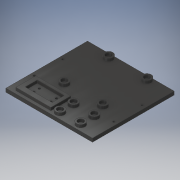
# Autodesk Inventor part: circuirt_board
Saved by Autodesk Inventor 2019 (Build 230136000, 136)
## iProperties
Created: 2018-11-27
Part Number: circuirt_board
Material: Generic
Document SubType Name: Modeling
Designer: xwermter
Density: 1 g/cm^3
Appearance: Default
Author: xwermter
Autodesk Inventor part; units mm, degrees
ref_plane "YZ Plane" through (0, 0, 0) normal (1, 0, 0) x (0, 1, 0)
ref_plane "XZ Plane" through (0, 0, 0) normal (0, 1, 0) x (-1, 0, 0)
ref_plane "XY Plane" through (0, 0, 0) normal (0, 0, 1) x (1, 0, 0)
sketch "Sketch1" plane through (0, 0, 0) normal (0, 1, 0) x (-1, 0, 0)
  line L0 (60.75, -57.25) -> (-60.75, -57.25)
  line L1 (-60.75, -57.25) -> (-60.75, 57.25)
  line L2 (-60.75, 57.25) -> (60.75, 57.25)
  line L3 (60.75, 57.25) -> (60.75, -57.25)
  line L4 (0, -80.15) -> (0, 80.15) projected
  line L5 (-85.05, 0) -> (85.05, 0) projected
  dimension "d0" = 121.5
  dimension "d1" = 114.5
  constraints: 8 end point, 2 parallel, 1 horizontal, 1 perpendicular, 2 other
  measures "d0" distance of L1.end L2.end
  measures "d1" distance of L0.end L1.end
extrude "Extrusion1" add sketch "Sketch1" along normal blind 5
sketch "Sketch3" plane through (0, 5, 0) normal (0, 1, 0) x (1, 0, 0)
  circle A0 centre (-36.75, -34.25) radius 1.5
  line L0 (-60.75, 57.25) -> (-60.75, -57.25) projected
  circle A1 centre (-12.75, -34.25) radius 1.5
  circle A2 centre (-36.75, -42.25) radius 1.5
  circle A3 centre (-12.75, -42.25) radius 1.5
  line L1 (-60.75, -57.25) -> (60.75, -57.25) projected
  circle A4 centre (-55.75, -22.25) radius 1.5
  circle A5 centre (-55.75, 17.75) radius 1.5
  circle A6 centre (-25.25, 51.25) radius 1.5
  circle A7 centre (28.75, 51.25) radius 1.5
  circle A8 centre (55.75, 17.75) radius 1.5
  circle A9 centre (55.75, -22.25) radius 1.5
  line L2 (60.75, 57.25) -> (-60.75, 57.25) projected
  line L3 (60.75, -57.25) -> (60.75, 57.25) projected
  circle A10 centre (-25.25, -10.75) radius 1.5
  circle A11 centre (28.75, -10.75) radius 1.5
  circle A12 centre (6.75, -29.75) radius 1.5
  circle A13 centre (6.75, -48.75) radius 1.5
  circle A14 centre (35.75, -48.75) radius 1.5
  circle A15 centre (35.75, -29.75) radius 1.5
  point P0 (0, 0)
  dimension "d11" = 3
  dimension "d12" = 24
  dimension "d13" = 3
  dimension "d14" = 3
  dimension "d15" = 3
  dimension "d16" = 24
  dimension "d17" = 24
  dimension "d20" = 23
  dimension "d21" = 23
  dimension "d22" = 8
  dimension "d23" = 8
  dimension "d24" = 15
  dimension "d25" = 3
  dimension "d26" = 3
  dimension "d27" = 5
  dimension "d28" = 5
  dimension "d29" = 35
  dimension "d30" = 40
  dimension "d31" = 3
  dimension "d32" = 3
  dimension "d33" = 3
  dimension "d34" = 3
  dimension "d35" = 6
  dimension "d36" = 6
  dimension "d37" = 5
  dimension "d38" = 5
  dimension "d39" = 35
  dimension "d40" = 40
  dimension "d41" = 32
  dimension "d42" = 54
  dimension "d43" = 3
  dimension "d44" = 3
  dimension "d45" = 62
  dimension "d46" = 62
  dimension "d47" = 54
  dimension "d48" = 32
  dimension "d49" = 3
  dimension "d50" = 3
  dimension "d51" = 3
  dimension "d52" = 3
  dimension "d53" = 8.5
  dimension "d54" = 8.5
  dimension "d55" = 25
  dimension "d56" = 29
  dimension "d57" = 19
  dimension "d58" = 19
  dimension "d59" = 25
  dimension "d60" = 29
  constraints: 16 centre point
  measures "d11" diameter of A0
  measures "d12" distance from line of L0 A0.centre
  measures "d13" diameter of A1
  measures "d14" diameter of A2
  measures "d15" diameter of A3
  measures "d16" distance of A1.centre A0.centre
  measures "d17" distance of A3.centre A2.centre
  measures "d20" distance from line of L1 A0.centre
  measures "d21" distance from line of L1 A1.centre
  measures "d22" distance of A0.centre A2.centre
  measures "d23" distance of A1.centre A3.centre
  measures "d24" distance from line of L1 A2.centre
  measures "d25" diameter of A4
  measures "d26" diameter of A5
  measures "d27" distance from line of L0 A5.centre
  measures "d28" distance from line of L0 A4.centre
  measures "d29" distance from line of L1 A4.centre
  measures "d30" distance of A4.centre A5.centre
  measures "d31" diameter of A6
  measures "d32" diameter of A7
  measures "d33" diameter of A8
  measures "d34" diameter of A9
  measures "d35" distance from line of L2 A6.centre
  measures "d36" distance from line of L2 A7.centre
  measures "d37" distance from line of L3 A8.centre
  measures "d38" distance from line of L3 A9.centre
  measures "d39" distance from line of L1 A9.centre
  measures "d40" distance of A8.centre A9.centre
  measures "d41" distance from line of L3 A7.centre
  measures "d42" distance of A6.centre A7.centre
  measures "d43" diameter of A10
  measures "d44" diameter of A11
  measures "d45" distance of A6.centre A10.centre
  measures "d46" distance of A11.centre A7.centre
  measures "d47" distance of A11.centre A10.centre
  measures "d48" distance from line of L3 A11.centre
  measures "d49" diameter of A12
  measures "d50" diameter of A13
  measures "d51" diameter of A14
  measures "d52" diameter of A15
  measures "d53" distance from line of L1 A13.centre
  measures "d54" distance from line of L1 A14.centre
  measures "d55" distance from line of L3 A14.centre
  measures "d56" distance of A13.centre A14.centre
  measures "d57" distance of A13.centre A12.centre
  measures "d58" distance of A14.centre A15.centre
  measures "d59" distance from line of L3 A15.centre
  measures "d60" distance of A15.centre A12.centre
extrude "Extrusion2" cut sketch "Sketch3" against normal through all contours A0 | A1 | A2 | A3 | A4 | A5 | A6 | A7 | A8 | A9 | A10 | A11 | A12 | A13 | A14 | A15
sketch "Sketch4" plane through (0, 5, 0) normal (0, 1, 0) x (1, 0, 0)
  line L0 (-44.75, -29.25) -> (-6.75, -29.25)
  line L1 (-6.75, -29.25) -> (-6.75, -46.25)
  line L2 (-6.75, -46.25) -> (-44.75, -46.25)
  line L3 (-44.75, -46.25) -> (-44.75, -29.25)
  line L4 (-50.75, -25.25) -> (-1.75, -25.25)
  line L5 (-1.75, -25.25) -> (-1.75, -53.25)
  line L6 (-1.75, -53.25) -> (-50.75, -53.25)
  line L7 (-50.75, -53.25) -> (-50.75, -25.25)
  line L8 (-60.75, 57.25) -> (-60.75, -57.25) projected
  line L9 (-60.75, -57.25) -> (60.75, -57.25) projected
  circle A0 centre (6.75, -29.75) radius 1.5 projected
  circle A1 centre (6.75, -29.75) radius 4
  circle A2 centre (6.75, -29.75) radius 6
  circle A3 centre (6.75, -48.75) radius 1.5 projected
  circle A4 centre (6.75, -48.75) radius 4
  circle A5 centre (6.75, -48.75) radius 6
  circle A6 centre (35.75, -29.75) radius 1.5 projected
  circle A7 centre (35.75, -29.75) radius 4
  circle A8 centre (35.75, -29.75) radius 6
  circle A9 centre (35.75, -48.75) radius 1.5 projected
  circle A10 centre (35.75, -48.75) radius 4
  circle A11 centre (35.75, -48.75) radius 6
  circle A12 centre (28.75, -10.75) radius 1.5 projected
  circle A13 centre (28.75, -10.75) radius 4
  circle A14 centre (28.75, -10.75) radius 6
  circle A15 centre (-25.25, -10.75) radius 1.5 projected
  circle A16 centre (-25.25, -10.75) radius 4
  circle A17 centre (-25.25, -10.75) radius 6
  circle A18 centre (-25.25, 51.25) radius 1.5 projected
  circle A19 centre (-25.25, 51.25) radius 4
  circle A20 centre (-25.25, 51.25) radius 6
  circle A21 centre (28.75, 51.25) radius 1.5 projected
  circle A22 centre (28.75, 51.25) radius 4
  circle A23 centre (28.75, 51.25) radius 6
  point P0 (0, 0)
  dimension "d63" = 49
  dimension "d64" = 28
  dimension "d71" = 5
  dimension "d72" = 4
  dimension "d73" = 6
  dimension "d74" = 7
  dimension "d75" = 59
  dimension "d76" = 32
  dimension "d77" = 8
  dimension "d78" = 12
  dimension "d79" = 8
  dimension "d80" = 12
  dimension "d81" = 8
  dimension "d82" = 12
  dimension "d83" = 8
  dimension "d84" = 12
  dimension "d85" = 8
  dimension "d86" = 12
  dimension "d87" = 8
  dimension "d88" = 12
  dimension "d89" = 8
  dimension "d90" = 12
  dimension "d91" = 8
  dimension "d92" = 12
  constraints: 16 centre point, 16 coincident, 16 end point, 4 parallel, 2 horizontal, 2 perpendicular
  measures "d63" distance of L4.start L4.end
  measures "d64" distance of L4.end L5.end
  measures "d71" distance between parallel lines of L5 L1
  measures "d72" distance between parallel lines of L4 L0
  measures "d73" distance between parallel lines of L7 L3
  measures "d74" distance between parallel lines of L2 L6
  measures "d75" distance between parallel lines of L5 L8
  measures "d76" distance between parallel lines of L9 L4
  measures "d77" diameter of A1
  measures "d78" diameter of A2
  measures "d79" diameter of A4
  measures "d80" diameter of A5
  measures "d81" diameter of A7
  measures "d82" diameter of A8
  measures "d83" diameter of A10
  measures "d84" diameter of A11
  measures "d85" diameter of A13
  measures "d86" diameter of A14
  measures "d87" diameter of A16
  measures "d88" diameter of A17
  measures "d89" diameter of A19
  measures "d90" diameter of A20
  measures "d91" diameter of A22
  measures "d92" diameter of A23
extrude "Extrusion3" add sketch "Sketch4" along normal blind 4 contours L4 L5 L6 L7 | A2 | A5 | A8 | A11 | A14 | A17 | A20 | A23
body "Solid1"
